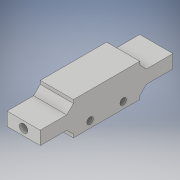
# Autodesk Inventor part: SliderSlider
Saved by Autodesk Inventor 2019 (Build 230136000, 136)
## iProperties
Created: 2019-10-06
Part Number: SliderSlider
Material: Generic
Document SubType Name: Modeling
Designer: james
Density: 1 g/cm^3
Appearance: Default
Author: james
Autodesk Inventor part; units mm, degrees
ref_plane "YZ Plane" through (0, 0, 0) normal (1, 0, 0) x (0, 1, 0)
ref_plane "XZ Plane" through (0, 0, 0) normal (0, 1, 0) x (-1, 0, 0)
ref_plane "XY Plane" through (0, 0, 0) normal (0, 0, 1) x (1, 0, 0)
sketch "Sketch1" plane through (0, 0, 0) normal (0, 0, 1) x (1, 0, 0)
  line L0 (-42.4234, 22.9681) -> (-17.0234, 22.9681)
  line L1 (-17.0234, 22.9681) -> (-17.0234, -2.4319)
  line L2 (-17.0234, -2.4319) -> (-42.4234, -2.4319)
  line L3 (-42.4234, -2.4319) -> (-42.4234, 22.9681)
  point P0 (0, 0)
  dimension "d0" = 25.4
  dimension "d1" = 25.4
  constraints: 8 end point, 2 parallel, 1 horizontal, 1 perpendicular
  measures "d0" distance of L1.end L2.end
  measures "d1" distance of L0.end L1.end
extrude "Extrusion1" add sketch "Sketch1" along normal blind 50.8
sketch "Sketch2" plane through (-17.0234, -2.4319, 0) normal (1, 0, 0) x (0, 0, -1)
  line L0 (-50.8, 22.86) -> (-50.8, 2.54)
  line L1 (-50.8, 2.54) -> (-55.88, 7.62)
  line L2 (-55.88, 7.62) -> (-76.2, 7.62)
  line L3 (-76.2, 7.62) -> (-76.2, 17.78)
  line L4 (-76.2, 17.78) -> (-55.88, 17.78)
  line L5 (-55.88, 17.78) -> (-50.8, 22.86)
  line L6 (-50.8, 0) -> (-50.8, 25.4) projected
  line L7 (0, 0) -> (-50.8, 0) projected
  point P0 (0, 2.4319)
  dimension "d4" = 25.4
  dimension "d5" = 20.32
  dimension "d6" = 5.08
  dimension "d7" = 5.08
  dimension "d8" = 5.08
  dimension "d9" = 5.08
  dimension "d10" = 0
  dimension "d11" = 2.54
  constraints: 12 end point, 3 perpendicular, 1 vertical
  measures "d4" distance between parallel lines of L0 L3
  measures "d5" distance of L0.start L0.end
  measures "d6" distance from line of L0.start L4
  measures "d7" horizontal distance of L0.end L1.end
  measures "d8" horizontal distance of L0.start L4.end
  measures "d9" horizontal distance of L0.end L1.end
  measures "d10" distance between parallel lines of L6 L0
  measures "d11" distance from line of L0.end L7
extrude "Extrusion2" add sketch "Sketch2" against normal blind 25.4
sketch "Sketch3" plane through (-17.0234, -2.4319, 0) normal (1, 0, 0) x (0, 0, -1)
  line L0 (0, 20.4965) -> (0, 2.54)
  line L1 (0, 2.54) -> (5.08, 7.62)
  line L2 (5.08, 7.62) -> (25.4, 7.62)
  line L3 (25.4, 7.62) -> (25.4, 17.78)
  line L4 (25.4, 17.78) -> (5.08, 17.78)
  line L5 (5.08, 17.78) -> (0, 22.86)
  line L6 (0, 22.86) -> (0, 20.4965)
  line L7 (-55.88, 7.62) -> (-76.2, 7.62) projected
  line L8 (-76.2, 17.78) -> (-55.88, 17.78) projected
  line L9 (0, 25.4) -> (0, 0) projected
  line L10 (0, 0) -> (-50.8, 0) projected
  point P0 (0, 2.4319)
  dimension "d14" = 20.32
  dimension "d15" = 5.08
  dimension "d16" = 5.08
  dimension "d17" = 5.08
  dimension "d18" = 5.08
  dimension "d19" = 25.4
  dimension "d20" = 10.16
  dimension "d21" = 0
  dimension "d22" = 2.54
  dimension "d23" = 10.16
  constraints: 14 end point, 3 perpendicular, 1 collinear, 1 point on line, 1 vertical
  measures "d14" distance of L0.end L5.end
  measures "d15" distance from line of L4 L5.end
  measures "d16" distance from line of L0.end L2
  measures "d17" distance from line of L0 L1.end
  measures "d18" horizontal distance of L5.end L4.end
  measures "d19" distance between parallel lines of L0 L3
  measures "d20" distance between parallel lines of L7 L8
  measures "d21" distance between parallel lines of L9 L0
  measures "d22" distance from line of L10 L0.end
  measures "d23" distance of L2.end L3.end
extrude "Extrusion3" add sketch "Sketch3" against normal blind 25.4
sketch "Sketch4" plane through (-17.0234, 5.1881, 76.2) normal (0, 0, 1) x (1, 0, 0)
  line L0 (0, 10.16) -> (-25.4, 10.16) projected
  line L1 (-25.4, 0) -> (-25.4, 10.16) projected
  point P0 (17.0234, -5.1881)
  point P1 (-12.7, 5.08)
  dimension "d26" = 5.08
  dimension "d27" = 12.7
  measures "d26" distance from line of point (-12.7, 5.08) L0
  measures "d27" distance from line of L1 point (-12.7, 5.08)
hole "Hole1" at (-29.7234, 10.2681, 76.2) direction (0, 0, -1) diameter 6.35 end through all
sketch "Sketch5" plane through (-17.0234, 22.9681, 50.8) normal (1, 0, 0) x (0, 0, -1)
  line L0 (50.8, -25.4) -> (0, -25.4) projected
  point P0 (50.8, -22.9681)
  point P1 (12.7, -20.32)
  point P2 (38.1, -20.32)
  dimension "d35" = 5.08
  dimension "d36" = 5.08
  dimension "d37" = 12.7
  dimension "d38" = 12.7
  measures "d35" distance from line of L0 point (38.1, -20.32)
  measures "d36" distance from line of L0 point (12.7, -20.32)
  measures "d37" horizontal distance of L0.end point (12.7, -20.32)
  measures "d38" horizontal distance of L0.start point (38.1, -20.32)
hole "Hole2" at (-17.0234, 2.6481, 38.1) at (-17.0234, 2.6481, 12.7) direction (-1, 0, 0) diameter 4.9784 end through all thread size "1/4-20 UNC" class "2B" standard "ANSI Unified Screw Threads"
body "Solid1"
